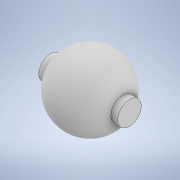
# Autodesk Inventor part: dragonfly_head
Saved by Autodesk Inventor 2021 (Build 250183000, 183)
## iProperties
Created: 2021-02-06
Part Number: dragonfly_head
Material: Generic
Document SubType Name: Modeling
Designer: dsdan
Density: 1 g/cm^3
Appearance: Default
Author: dsdan
Autodesk Inventor part; units mm, degrees
ref_plane "YZ Plane" through (0, 0, 0) normal (1, 0, 0) x (0, 1, 0)
ref_plane "XZ Plane" through (0, 0, 0) normal (0, 1, 0) x (-1, 0, 0)
ref_plane "XY Plane" through (0, 0, 0) normal (0, 0, 1) x (1, 0, 0)
sketch "Sketch1" plane through (0, 0, 0) normal (0, 1, 0) x (-1, 0, 0)
  circle A0 centre (0, 0) radius 5
  line L0 (-5.7156, -1.6905) -> (5.7156, -1.6905)
  line L1 (5.7156, -1.6905) -> (5.7156, 1.6905)
  line L2 (5.7156, 1.6905) -> (-5.7156, 1.6905)
  line L3 (-5.7156, 1.6905) -> (-5.7156, -1.6905)
  line L4 (-5.7156, -1.6905) -> (5.7156, 1.6905) construction
  line L5 (5.7156, -1.6905) -> (-5.7156, 1.6905) construction
  line L6 (5.7156, 0) -> (-5.7156, 0)
  point P0 (5, 0)
  point P1 (-5, 0)
  point P2 (4.7055, 1.6905)
  point P3 (-4.7055, 1.6905)
  dimension "d0" = 10
  constraints: 14 end point, 4 midpoint, 2 parallel, 2 point on circle, 1 centre point, 1 coincident, 1 perpendicular
  measures "d0" diameter of A0
revolve "Revolution1" add sketch "Sketch1" angle 360 about axis through (-5.7156, 0, 0) along (1, 0, 0) contours L6 A0 L2 | A0 L2 L1 L6 | L2 A0 | L6 L3 L2 A0
body "Solid1"
